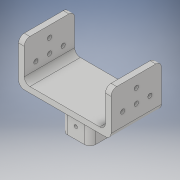
# Autodesk Inventor part: Drone_holder_base
Saved by Autodesk Inventor 2019 (Build 230136000, 136)
## iProperties
Created: 2020-01-24
Part Number: Drone_holder_base
Material: Generic
Document SubType Name: Modeling
Designer: Next
Density: 1 g/cm^3
Appearance: Default
Author: Next
## iProperties of the stored document Drone_holder_base_3DPrint.ipt
Created: 2020-01-31
Part Number: Drone_holder_base_3DPrint
Material: Generic
Document SubType Name: Modeling
Designer: Next
Density: 1 g/cm^3
Appearance: Default
Author: Next
Autodesk Inventor part; units mm, degrees
ref_plane "YZ Plane" through (0, 0, 0) normal (1, 0, 0) x (0, 1, 0)
ref_plane "XZ Plane" through (0, 0, 0) normal (0, 1, 0) x (-1, 0, 0)
ref_plane "XY Plane" through (0, 0, 0) normal (0, 0, 1) x (1, 0, 0)
sketch "Sketch1" plane through (0, 0, 0) normal (0, 1, 0) x (-1, 0, 0)
  line L0 (0, 0) -> (-98, 0)
  line L1 (-98, 0) -> (-98, -53.377)
  line L2 (-98, -53.377) -> (0, -53.377)
  line L3 (0, -53.377) -> (0, 0)
  line L4 (-98, -53.377) -> (0, 0) construction
  dimension "d0" = 98
  dimension "d1" = 53.377
  constraints: 10 end point, 2 parallel, 1 horizontal, 1 perpendicular
  measures "d0" distance of L2.end L1.end
  measures "d1" distance of L1.end L0.end
extrude "Extrusion1" add sketch "Sketch1" along normal blind 6
sketch "Sketch2" plane through (0, 6, 0) normal (0, 1, 0) x (1, 0, 0)
  line L0 (98, 0) -> (98, 53.377) projected
  line L1 (0, 0) -> (98, 0) projected
  line L2 (98, 53.377) -> (92, 53.377)
  line L3 (92, 53.377) -> (92, 0)
  line L4 (92, 0) -> (98, 0)
  line L5 (98, 0) -> (98, 53.377)
  line L6 (0, 53.377) -> (6, 53.377)
  line L7 (6, 53.377) -> (6, 0)
  line L8 (6, 0) -> (0, 0)
  line L9 (0, 0) -> (0, 53.377)
  dimension "d4" = 6
  dimension "d5" = 6
  constraints: 16 end point, 4 parallel, 3 point on line, 2 horizontal, 2 perpendicular
  measures "d4" distance of L4.end L3.end
  measures "d5" distance of L7.end L8.end
extrude "Extrusion2" add sketch "Sketch2" along normal blind 40
sketch "Sketch3" plane through (0, 0, -53.377) normal (-1, 0, 0) x (0, 0, 1)
  arc A0 (41.0993, 20) -> (12.1996, 20) centre (26.6494, 20.0723) ccw construction
  arc A1 (43.3493, 19.9888) -> (9.9496, 19.9888) centre (26.6494, 20.0723) ccw
  arc A2 (38.8493, 20.0113) -> (14.4496, 20.0113) centre (26.6494, 20.0723) ccw
  arc A3 (38.8493, 20.0113) -> (43.3493, 19.9888) centre (41.0993, 20) ccw
  arc A4 (9.9496, 19.9888) -> (14.4496, 20.0113) centre (12.1996, 20) ccw
  circle A5 centre (26.6495, 20) radius 2.25
  circle A6 centre (41.0993, 20) radius 2.25
  circle A7 centre (12.1996, 20) radius 2.25
  circle A8 centre (26.6494, 34.5224) radius 2.25
  point P0 (53.377, 0)
  dimension "d8" = 4.5
  dimension "d9" = 4.5
  dimension "d36" = 14.45
  constraints: 11 point on circle, 9 centre point, 5 tangent, 3 coincident, 2 concentric
  measures "d8" diameter of A3
  measures "d9" diameter of A5
  measures "d36" radius of A0
extrude "Extrusion3" cut sketch "Sketch3" against normal blind 110 and the other way blind 12.5 contours A3 A6 A1 | A8 | A7 A4 | A5
sketch "Sketch4" plane through (0, 0, 0) normal (0, -1, 0) x (1, 0, 0)
  line L0 (98, -53.377) -> (92, -53.377) construction
  line L1 (98, -53.377) -> (0, 0) construction
  line L2 (64, -41.6885) -> (34, -41.6885)
  line L3 (34, -41.6885) -> (34, -11.6885)
  line L4 (34, -11.6885) -> (64, -11.6885)
  line L5 (64, -11.6885) -> (64, -41.6885)
  line L6 (64, -41.6885) -> (34, -11.6885) construction
  line L7 (34, -41.6885) -> (64, -11.6885) construction
  circle A0 centre (49, -26.6885) radius 11.75
  dimension "d16" = 30
  dimension "d17" = 30
  dimension "d18" = 23.5
  constraints: 14 end point, 3 midpoint, 2 parallel, 1 centre point, 1 coincident, 1 horizontal, 1 perpendicular
  measures "d16" distance of L3.end L4.end
  measures "d17" distance of L2.end L3.end
  measures "d18" diameter of A0
extrude "Extrusion4" add sketch "Sketch4" along normal blind 30
sketch "Sketch5" plane through (34, 0, -11.6885) normal (0, 0, 1) x (1, 0, 0)
  line L0 (0, -30) -> (30, -30) construction
  line L1 (30, 0) -> (0, 0) construction
  circle A0 centre (15, -18) radius 1.75
  point P0 (-34, 0)
  dimension "d21" = 3.5
  dimension "d26" = 12
  constraints: 1 centre point
  measures "d21" diameter of A0
  measures "d26" distance from line of L0 A0.centre
extrude "Extrusion5" cut sketch "Sketch5" against normal blind 33
sketch "Sketch7" plane through (34, 0, -41.6885) normal (-1, 0, 0) x (0, 0, 1)
  line L0 (0, 0) -> (0, -30) construction
  line L1 (30, 0) -> (30, -30) construction
  circle A0 centre (15, -18) radius 1.75
  line L2 (30, -30) -> (0, -30) projected
  point P0 (41.6885, 0)
  dimension "d31" = 3.5
  dimension "d32" = 12
  constraints: 1 centre point
  measures "d31" diameter of A0
  measures "d32" distance from line of L2 A0.centre
extrude "Extrusion7" cut sketch "Sketch7" against normal blind 33
fillet "Fillet3" radius 6 16 edges at (0, 0, -26.6885) (98, 0, -26.6885) (64, -15, -41.6885) (34, -15, -41.6885) (49, 0, -41.6885) (34, 0, -26.6885) (34, -15, -11.6885) (49, 0, -11.6885) (64, -15, -11.6885) (64, 0, -26.6885) (6, 6, -26.6885) (92, 6, -26.6885) (95, 46, 0) (3, 46, 0) (3, 46, -53.377) (95, 46, -53.377)
body "Solid1"
